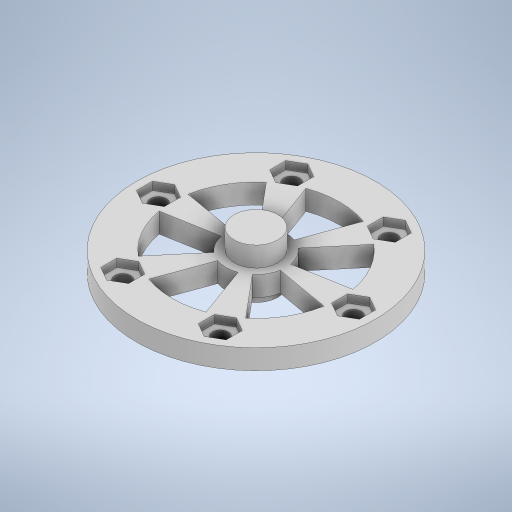
# Autodesk Inventor part: Reaction_wheel
Saved by Autodesk Inventor 2023 (Build 270158000, 158)
## iProperties
Created: 2022-12-10
Part Number: Reaction_wheel
Material: Generic
Document SubType Name: Modeling
Designer: Krzysztof
Density: 1 g/cm^3
Appearance: Default
Mass: 80.311 g
Surface Area: 283.825 cm^2
Volume: 80.311 cm^3
Author: Krzysztof
Autodesk Inventor part; units mm, degrees
ref_plane "YZ Plane" through (0, 0, 0) normal (1, 0, 0) x (0, 1, 0)
ref_plane "XZ Plane" through (0, 0, 0) normal (0, 1, 0) x (-1, 0, 0)
ref_plane "XY Plane" through (0, 0, 0) normal (0, 0, 1) x (1, 0, 0)
sketch "Sketch1" plane through (0, 0, 0) normal (0, 1, 0) x (-1, 0, 0)
  circle A0 centre (0, 0) radius 60
  line L0 (14.7721, 2.6047) -> (41.3619, 7.2932)
  line L1 (14.7721, -2.6047) -> (41.3619, -7.2932)
  line L2 (0, 0) -> (115.9423, 0) construction
  line L3 (0, 0) -> (87.3255, -15.3978) construction
  line L4 (5.1303, 14.0954) -> (14.3648, 39.4671)
  line L5 (9.6418, 11.4907) -> (26.9971, 32.1739)
  line L6 (-9.6418, 11.4907) -> (-26.9971, 32.1739)
  line L7 (-5.1303, 14.0954) -> (-14.3648, 39.4671)
  line L8 (-14.7721, -2.6047) -> (-41.3619, -7.2932)
  line L9 (-14.7721, 2.6047) -> (-41.3619, 7.2932)
  line L10 (-5.1303, -14.0954) -> (-14.3648, -39.4671)
  line L11 (-9.6418, -11.4907) -> (-26.9971, -32.1739)
  line L12 (9.6418, -11.4907) -> (26.9971, -32.1739)
  line L13 (5.1303, -14.0954) -> (14.3648, -39.4671)
  arc A1 (41.3619, 7.2932) -> (26.9971, 32.1739) centre (0, 0) ccw
  arc A2 (26.9971, -32.1739) -> (41.3619, -7.2932) centre (0, 0) ccw
  arc A3 (-14.3648, -39.4671) -> (14.3648, -39.4671) centre (0, 0) ccw
  arc A4 (-41.3619, -7.2932) -> (-26.9971, -32.1739) centre (0, 0) ccw
  arc A5 (14.3648, 39.4671) -> (-14.3648, 39.4671) centre (0, 0) ccw
  arc A6 (-26.9971, 32.1739) -> (-41.3619, 7.2932) centre (0, 0) ccw
  circle A7 centre (0, 0) radius 42 construction
  circle A8 centre (0, 0) radius 15 construction
  arc A9 (9.6418, -11.4907) -> (14.7721, -2.6047) centre (0, 0) ccw
  arc A10 (-5.1303, -14.0954) -> (5.1303, -14.0954) centre (0, 0) ccw
  arc A11 (-14.7721, -2.6047) -> (-9.6418, -11.4907) centre (0, 0) ccw
  arc A12 (-9.6418, 11.4907) -> (-14.7721, 2.6047) centre (0, 0) ccw
  arc A13 (14.7721, 2.6047) -> (9.6418, 11.4907) centre (0, 0) ccw
  arc A14 (5.1303, 14.0954) -> (-5.1303, 14.0954) centre (0, 0) ccw
  dimension "d12" = 30
  dimension "d13" = 84
  dimension "d0" = 120
  dimension "d3" = 20
  dimension "d4" = 10
  dimension "d10" = 360
  constraints: 28 end point, 24 point on circle, 13 centre point, 5 coincident, 1 horizontal, 1 point on line, 44 other
  measures "d0" diameter of A0
  measures "d3" angle of L1 L0
  measures "d4" angle of L2 L3
extrude "Extrusion1" add sketch "Sketch1" against normal blind 10
sketch "Sketch2" plane through (0, 0, 0) normal (0, 1, 0) x (1, 0, 0)
  circle A0 centre (-49, 0) radius 4
  line L0 (0, 0) -> (-95.2262, 0) construction
  line L1 (-49, 8.0829) -> (-42, 4.0415)
  line L2 (-42, 4.0415) -> (-42, -4.0415)
  line L3 (-42, -4.0415) -> (-49, -8.0829)
  line L4 (-49, -8.0829) -> (-56, -4.0415)
  line L5 (-56, -4.0415) -> (-56, 4.0415)
  line L6 (-56, 4.0415) -> (-49, 8.0829)
  line L7 (0, 0) -> (0, 100.6491) construction
  circle A1 centre (-24.5, -42.4352) radius 4
  line L8 (-31.5, -38.3938) -> (-24.5, -34.3523)
  line L9 (-24.5, -34.3523) -> (-17.5, -38.3938)
  line L10 (-17.5, -38.3938) -> (-17.5, -46.4767)
  line L11 (-17.5, -46.4767) -> (-24.5, -50.5181)
  line L12 (-24.5, -50.5181) -> (-31.5, -46.4767)
  line L13 (-31.5, -46.4767) -> (-31.5, -38.3938)
  circle A2 centre (24.5, -42.4352) radius 4
  line L14 (17.5, -46.4767) -> (17.5, -38.3938)
  line L15 (17.5, -38.3938) -> (24.5, -34.3523)
  line L16 (24.5, -34.3523) -> (31.5, -38.3938)
  line L17 (31.5, -38.3938) -> (31.5, -46.4767)
  line L18 (31.5, -46.4767) -> (24.5, -50.5181)
  line L19 (24.5, -50.5181) -> (17.5, -46.4767)
  circle A3 centre (49, 0) radius 4
  line L20 (49, -8.0829) -> (42, -4.0415)
  line L21 (42, -4.0415) -> (42, 4.0415)
  line L22 (42, 4.0415) -> (49, 8.0829)
  line L23 (49, 8.0829) -> (56, 4.0415)
  line L24 (56, 4.0415) -> (56, -4.0415)
  line L25 (56, -4.0415) -> (49, -8.0829)
  circle A4 centre (24.5, 42.4352) radius 4
  line L26 (31.5, 38.3938) -> (24.5, 34.3523)
  line L27 (24.5, 34.3523) -> (17.5, 38.3938)
  line L28 (17.5, 38.3938) -> (17.5, 46.4767)
  line L29 (17.5, 46.4767) -> (24.5, 50.5181)
  line L30 (24.5, 50.5181) -> (31.5, 46.4767)
  line L31 (31.5, 46.4767) -> (31.5, 38.3938)
  circle A5 centre (-24.5, 42.4352) radius 4
  line L32 (-17.5, 46.4767) -> (-17.5, 38.3938)
  line L33 (-17.5, 38.3938) -> (-24.5, 34.3523)
  line L34 (-24.5, 34.3523) -> (-31.5, 38.3938)
  line L35 (-31.5, 38.3938) -> (-31.5, 46.4767)
  line L36 (-31.5, 46.4767) -> (-24.5, 50.5181)
  line L37 (-24.5, 50.5181) -> (-17.5, 46.4767)
  dimension "d16" = 8
  dimension "d17" = 49
  dimension "d18" = 14
  dimension "d21" = 360
  constraints: 76 end point, 6 centre point, 6 coincident, 1 horizontal, 1 parallel, 1 point on line, 1 vertical, 104 other
  measures "d16" diameter of A0
  measures "d17" distance of L0.start A0.centre
  measures "d18" distance between parallel lines of L3 L6
extrude "Extrusion2" cut sketch "Sketch2" against normal blind 4 contours A0 | L1 L2 L3 L4 L5 L6 | A1 | L8 L9 L10 L11 L12 L13 | A2 | L14 L15 L16 L17 L18 L19 | A3 | L20 L21 L22 L23 L24 L25 | A4 | L26 L27 L28 L29 L30 L31 | A5 | L32 L33 L34 L35 L36 L37
extrude "Extrusion3" cut sketch "Sketch2" against normal through all contours A0 | A1 | A2 | A3 | A4 | A5
sketch "Sketch3" plane through (0, -10, 0) normal (0, -1, 0) x (1, 0, 0)
  circle A0 centre (0, 0) radius 11
  dimension "d27" = 22
  constraints: 1 centre point, 1 coincident
  measures "d27" diameter of A0
extrude "Extrusion4" add sketch "Sketch3" along normal blind 5 and the other way blind 20
sketch "Sketch4" plane through (0, -15, 0) normal (0, -1, 0) x (1, 0, 0)
  arc A0 (-1.5, 2) -> (1.5, 2) centre (0, 0) ccw
  line L0 (-1.5, 2) -> (1.5, 2)
  dimension "d30" = 5
  dimension "d31" = 2
  constraints: 2 end point, 2 point on circle, 1 centre point, 1 coincident, 1 horizontal
  measures "d30" diameter of A0
  measures "d31" distance from line of L0 A0.centre
extrude "Extrusion5" cut sketch "Sketch4" against normal blind 20
body "Solid1"
